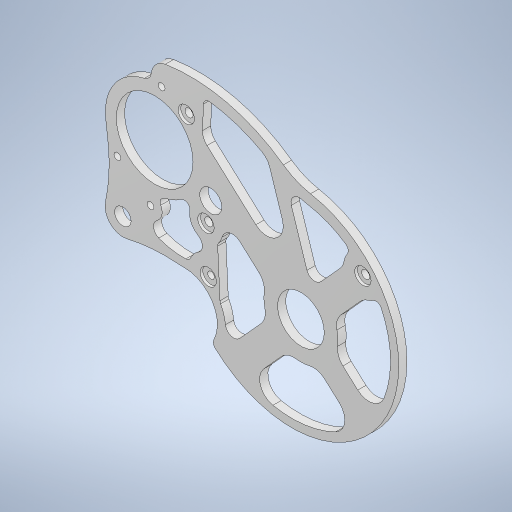
# Autodesk Inventor part: 足内フレーム
Saved by Autodesk Inventor 2023 (Build 270158000, 158)
## iProperties
Created: 2022-01-10
Part Number: 足内フレーム
Material: Aluminum 2014-T4
Document SubType Name: Modeling
Designer: acps
Density: 2.8 g/cm^3
Appearance: Satin
Author: acps
Autodesk Inventor part; units mm, degrees
ref_plane "YZ Plane" through (0, 0, 0) normal (1, 0, 0) x (0, 1, 0)
ref_plane "XZ Plane" through (0, 0, 0) normal (0, 1, 0) x (-1, 0, 0)
ref_plane "XY Plane" through (0, 0, 0) normal (0, 0, 1) x (1, 0, 0)
sketch "Sketch9" plane through (0, 0, 0) normal (0, 0, 1) x (1, 0, 0)
  circle A0 centre (46.616, 30) radius 14
  circle A1 centre (67.0906, 21) radius 20.5 construction
  arc A2 (89.1412, -35.261) -> (103.4815, 41.4054) centre (96.6972, 3) ccw
  arc A3 (28.8489, 27.1141) -> (89.1412, -35.261) centre (103.8658, 39.2989) ccw construction
  arc A4 (68.1999, -22.3859) -> (57.3086, -4.9334) centre (57.511, -16.9317) ccw
  arc A5 (68.1999, -22.3859) -> (68.6165, -24.7568) centre (69.9813, -23.2949) ccw
  arc A6 (68.6165, -24.7568) -> (89.1412, -35.261) centre (97.2785, 5.9432) ccw
  circle A7 centre (65.359, 13) radius 3
  circle A8 centre (66.1789, -3.483) radius 4 construction
  circle A9 centre (66.1789, -3.483) radius 3
  circle A10 centre (66.1789, -3.483) radius 1.25
  circle A11 centre (49.1519, 48.073) radius 1.25
  circle A12 centre (45.1, 8.5) radius 1.25
  circle A13 centre (33, 18) radius 1.25
  arc A14 (110.5809, -8.3302) -> (32.9301, 51.0574) centre (65.359, 13) ccw construction
  circle A15 centre (65.359, 13) radius 1.5
  arc A16 (116.9346, 29.0833) -> (126.4034, 19.1104) centre (122.6202, 25) ccw
  arc A17 (129.2953, 18.2763) -> (126.4034, 19.1104) centre (127.4843, 17.4276) ccw
  arc A18 (116.9346, 29.0833) -> (116.4381, 31.9015) centre (115.3101, 30.25) ccw
  circle A19 centre (67.0906, 21) radius 1.5
  circle A20 centre (67.0906, 21) radius 4.5 construction
  circle A21 centre (49.1519, 48.073) radius 4.25 construction
  arc A22 (42.888, 47.6097) -> (45.3636, 50.3845) centre (42.2376, 50.6816) ccw
  arc A23 (42.888, 47.6097) -> (28.8489, 27.1141) centre (46.616, 30) ccw
  arc A24 (50.502, 55.8582) -> (45.3636, 50.3845) centre (51.4661, 49.8045) ccw
  arc A25 (93.5981, 45.5879) -> (50.502, 55.8582) centre (59.6238, -1.42) ccw
  arc A26 (93.5981, 45.5879) -> (103.4815, 41.4054) centre (107.6564, 65.0395) ccw
  arc A27 (116.4381, 31.9015) -> (102.7857, 37.4664) centre (96.6972, 3) ccw
  arc A28 (91.2551, 42.346) -> (102.7857, 37.4664) centre (107.6564, 65.0395) ccw
  arc A29 (91.2551, 42.346) -> (66.6678, 52.1186) centre (59.6238, -1.42) ccw
  arc A30 (66.6678, 52.1186) -> (64.4084, 50.2128) centre (66.4069, 50.1357) ccw
  line L0 (64.4084, 50.2128) -> (63.6467, 30.4665)
  arc A31 (63.6467, 30.4665) -> (65.9495, 28.4127) centre (65.6452, 30.3894) ccw
  arc A32 (72.0057, 15.3351) -> (65.9495, 28.4127) centre (67.0906, 21) ccw
  arc A33 (62.3527, 39.5241) -> (63.2626, 46.965) centre (58.1571, 43.8132) ccw construction
  arc A34 (72.0057, 15.3351) -> (71.327, 13.6183) centre (73.3164, 13.8244) ccw
  arc A35 (70.0506, 9.2598) -> (71.327, 13.6183) centre (65.359, 13) ccw
  arc A36 (63.4085, 27.3516) -> (62.8815, 34.943) centre (46.616, 30) ccw construction
  arc A37 (70.0506, 9.2598) -> (69.6169, 7.9138) centre (71.6145, 8.0131) ccw
  line L1 (69.6169, 7.9138) -> (70.4543, -8.9212)
  arc A38 (70.4543, -8.9212) -> (70.6941, -9.7759) centre (72.4519, -8.8218) ccw
  arc A39 (71.6917, -21.8214) -> (70.6941, -9.7759) centre (57.511, -16.9317) ccw
  arc A40 (72.3015, -24.0094) -> (89.7225, -32.3179) centre (97.2785, 5.9432) ccw
  arc A41 (71.6917, -21.8214) -> (72.3015, -24.0094) centre (73.5824, -22.4733) ccw
  line L2 (65.359, 13) -> (66.1789, -3.483) construction
  arc A42 (89.7225, -32.3179) -> (129.2953, 18.2763) centre (96.6972, 3) ccw
  arc A43 (29.8136, 19.0227) -> (57.3086, -4.9334) centre (56.8493, 22.2958) ccw
  arc A44 (50.2005, 13.3822) -> (56.3412, 16.0565) centre (46.616, 30) ccw
  arc A45 (59.4537, 14.062) -> (56.3412, 16.0565) centre (57.4853, 14.4161) ccw
  arc A46 (47.4858, 4.9828) -> (48.8551, 10.4905) centre (45.1, 8.5) ccw
  arc A47 (59.4537, 14.062) -> (62.4846, 7.7333) centre (65.359, 13) ccw
  arc A48 (48.0848, -0.2968) -> (58.0139, -1.9093) centre (56.8493, 22.2958) ccw
  arc A49 (62.5868, 2.5251) -> (59.7536, -0.7053) centre (66.1789, -3.483) ccw
  arc A50 (58.0139, -1.9093) -> (59.7536, -0.7053) centre (57.9178, 0.0884) ccw
  arc A51 (50.2005, 13.3822) -> (48.8551, 10.4905) centre (50.6222, 11.4271) ccw
  arc A52 (62.5868, 2.5251) -> (62.4846, 7.7333) centre (61.0474, 5.1) ccw
  arc A53 (47.4858, 4.9828) -> (48.0848, -0.2968) centre (49.1698, 2.5001) ccw
  circle A54 centre (33, 18) radius 3 construction
  line L3 (29.8136, 19.0227) -> (28.7465, 27.8366)
  circle A55 centre (122.6202, 25) radius 3
  circle A56 centre (122.6202, 25) radius 1.5
  circle A57 centre (100, 0) radius 30 construction
  circle A58 centre (100, 0) radius 8.525
  circle A59 centre (100, 0) radius 13.525
  circle A60 centre (58.1571, 43.8132) radius 3
  circle A61 centre (58.1571, 43.8132) radius 1.5
  arc A62 (114.2643, 23.2173) -> (115.7252, 26.2077) centre (109.8151, 27.2429) ccw
  line L4 (114.2643, 23.2173) -> (107.1156, 15.3165)
  arc A63 (101.847, 13.3983) -> (107.1156, 15.3165) centre (102.6664, 19.3421) ccw
  line L5 (100, 0) -> (122.6202, 25) construction
  arc A64 (124.5093, 18.2597) -> (121.6794, 16.5079) centre (126.1286, 12.4824) ccw
  arc A65 (114.5307, 8.6072) -> (113.1474, 3.1737) centre (118.9799, 4.5816) ccw
  line L6 (114.5307, 8.6072) -> (121.6794, 16.5079)
  line L7 (100, 0) -> (74.2211, 23.325) construction
  arc A66 (91.3928, 14.5307) -> (96.8263, 13.1474) centre (95.4184, 18.9799) ccw
  arc A67 (86.6017, 1.847) -> (84.6835, 7.1156) centre (80.6579, 2.6664) ccw
  line L8 (77.7137, 13.4219) -> (84.6835, 7.1156)
  line L9 (91.3928, 14.5307) -> (65.7201, 37.7597)
  arc A68 (77.7137, 13.4219) -> (71.1616, 11.4735) centre (75.0299, 10.4559) ccw
  arc A69 (64.0785, 41.66) -> (65.7201, 37.7597) centre (69.0748, 41.4673) ccw
  arc A70 (108.6072, -14.5307) -> (103.1737, -13.1474) centre (104.5816, -18.9799) ccw
  arc A71 (113.3983, -1.847) -> (115.3165, -7.1156) centre (119.3421, -2.6664) ccw
  line L10 (100, 0) -> (122.2456, -20.128) construction
  line L11 (108.6072, -14.5307) -> (114.0305, -19.4378)
  line L12 (115.3165, -7.1156) -> (120.7448, -12.0272)
  arc A72 (112.6664, -29.2643) -> (114.0305, -19.4378) centre (110.0049, -23.8869) ccw
  arc A73 (120.7448, -12.0272) -> (130.3851, -9.6937) centre (124.7704, -7.5781) ccw
  arc A74 (85.4693, -8.6072) -> (86.8526, -3.1737) centre (81.0201, -4.5816) ccw
  arc A75 (98.153, -13.3983) -> (92.8844, -15.3165) centre (97.3336, -19.3421) ccw
  line L13 (85.4693, -8.6072) -> (77.655, -17.2435)
  line L14 (86.4647, -22.4117) -> (92.8844, -15.3165)
  line L15 (100, 0) -> (77.6565, -24.6942) construction
  arc A76 (72.4439, -15.5142) -> (77.655, -17.2435) centre (75.4304, -15.2307) ccw
  arc A77 (86.4647, -22.4117) -> (89.7566, -32.3246) centre (90.9138, -26.4372) ccw
  line L16 (93.2749, 27.9268) -> (88.6115, 42.3986)
  arc A78 (88.6115, 42.3986) -> (85.8103, 45.8057) centre (82.9007, 40.5584) ccw
  line L17 (102.1859, 16.5753) -> (96.489, 34.2545)
  arc A79 (100.1488, 38.0647) -> (96.489, 34.2545) centre (99.3445, 35.1746) ccw
  line L18 (91.2551, 42.346) -> (98.5171, 19.8098) construction
  arc A80 (102.1859, 16.5753) -> (107.2659, 15.4827) centre (105.0414, 17.4955) ccw
  arc A81 (83.5385, 21.6375) -> (93.2749, 27.9268) centre (87.5641, 26.0866) ccw
  circle A82 centre (67.0906, 21) radius 4.025
  circle A83 centre (35, 0) radius 3.025
  circle A84 centre (35, 0) radius 6.5
  arc A85 (28.6471, 1.3751) -> (29.7376, 19.7272) centre (-29.9949, 14.0681) ccw
  arc A86 (54.8296, -4.8623) -> (36.5033, -6.3238) centre (50.3798, -64.6971) ccw
  point P0 (0, 0)
  point P1 (0, 0)
  point P2 (89.7528, -32.3239)
  point P3 (89.7566, -32.3246)
  point P4 (29.7671, 19.4073)
  dimension "d291" = 2
  dimension "d292" = 42
  dimension "d293" = 74
  dimension "d294" = 118
  dimension "d295" = 6
  dimension "d296" = 8
  dimension "d297" = 6
  dimension "d298" = 2.5
  dimension "d299" = 2.5
  dimension "d300" = 2.5
  dimension "d301" = 8.5
  dimension "d302" = 45.1
  dimension "d303" = 2.5
  dimension "d304" = 18
  dimension "d305" = 33
  dimension "d306" = 50
  dimension "d307" = 3
  dimension "d308" = 2
  dimension "d309" = 2
  dimension "d310" = 3
  dimension "d311" = 3
  dimension "d312" = 3
  dimension "d313" = 4
  dimension "d314" = 4
  dimension "d315" = 2
  dimension "d316" = 2
  dimension "d317" = 3
  dimension "d318" = 2
  dimension "d319" = 3
  dimension "d320" = 3
  dimension "d321" = 2
  dimension "d322" = 2
  dimension "d323" = 3
  dimension "d324" = 2
  dimension "d325" = 3
  dimension "d326" = 12
  dimension "d327" = 3
  dimension "d328" = 2
  dimension "d329" = 3
  dimension "d330" = 3
  dimension "d331" = 3
  dimension "d332" = 3
  dimension "d333" = 2
  dimension "d334" = 3
  dimension "d335" = 3
  dimension "d336" = 2
  dimension "d337" = 6
  dimension "d338" = 4
  dimension "d339" = 17.05
  dimension "d340" = 5
  dimension "d341" = 3
  dimension "d342" = 6
  dimension "d343" = 6
  dimension "d344" = 5
  dimension "d345" = 6
  dimension "d346" = 6
  dimension "d347" = 10
  dimension "d348" = 6
  dimension "d349" = 6
  dimension "d350" = 10
  dimension "d351" = 5
  dimension "d352" = 4
  dimension "d353" = 5
  dimension "d354" = 6
  constraints: 141 point on circle, 85 centre point, 77 tangent, 38 end point, 14 concentric, 11 parallel, 9 coincident, 3 perpendicular, 3 point on line, 1 horizontal alignment, 39 other
  measures "d291" radius of A5
  measures "d292" radius of A6
  measures "d295" diameter of A7
  measures "d296" diameter of A8
  measures "d297" diameter of A9
  measures "d298" diameter of A10
  measures "d299" diameter of A11
  measures "d300" diameter of A12
  measures "d301" vertical distance of point (0, 0) A12.centre
  measures "d302" horizontal distance of point (0, 0) A12.centre
  measures "d303" diameter of A13
  measures "d304" vertical distance of point (0, 0) A13.centre
  measures "d305" horizontal distance of point (0, 0) A13.centre
  measures "d306" radius of A14
  measures "d307" diameter of A15
  measures "d308" radius of A17
  measures "d309" radius of A18
  measures "d310" diameter of A19
  measures "d311" radial gap between concentric circles of A19 A20
  measures "d312" radial gap between concentric circles of A11 A21
  measures "d313" radial gap between concentric circles of A27 A2
  measures "d314" radial gap between concentric circles of A28 A26
  measures "d315" radius of A30
  measures "d316" radius of A31
  measures "d317" radial gap between concentric circles of A20 A32
  measures "d318" radius of A34
  measures "d319" radial gap between concentric circles of A7 A35
  measures "d320" radial gap between concentric circles of A0 A36
  measures "d321" radius of A37
  measures "d322" radius of A38
  measures "d323" radial gap between concentric circles of A4 A39
  measures "d324" radius of A41
  measures "d325" radial gap between concentric circles of A2 A42
  measures "d326" radius of A4
  measures "d327" radial gap between concentric circles of A0 A44
  measures "d328" radius of A45
  measures "d329" radial gap between concentric circles of A12 A46
  measures "d330" radial gap between concentric circles of A7 A47
  measures "d331" radial gap between concentric circles of A43 A48
  measures "d332" radial gap between concentric circles of A49 A8
  measures "d333" radius of A51
  measures "d334" radius of A52
  measures "d335" radius of A53
  measures "d336" radius of A50
  measures "d337" diameter of A54
  measures "d338" radial gap between concentric circles of A16 A55
  measures "d339" diameter of A58
  measures "d341" radial gap between concentric circles of A33 A60
  measures "d342" radius of A62
  measures "d343" radius of A63
  measures "d344" distance between parallel lines of L5 L4
  measures "d345" radius of A64
  measures "d346" radius of A65
  measures "d347" distance between parallel lines of L4 L6
  measures "d348" radius of A66
  measures "d349" radius of A67
  measures "d350" distance between parallel lines of L8 L9
  measures "d351" distance between parallel lines of L9 L7
  measures "d352" radius of A68
  measures "d353" radius of A69
  measures "d354" radius of A70
extrude "Extrusion6" add sketch "Sketch9" along normal blind 3 contours A6 A5 A4 A43 A84 L3 A23 A22 A24 A25 A26 A2 | A86 A84 A43 | A84 A43 | A43 A84 | A84 A85 L3 A43 | A16 A64 L6 A65 A59 A63 L4 A62 | L4 A63 A59 A66 L9 A81 L16 A78 A29 A28 A79 L17 A80 | A42 A72 L11 A70 A59 A71 L12 A73 | A59 | A59 A67 L8 A68 A35 A34 A32 A31 L0 A69 L9 A66 | A40 A41 A39 A76 L13 A74 A59 A75 L14 A77
extrude "Extrusion7" add sketch "Sketch9" along normal blind 2 contours A7 | A9 | A55 | A60
sketch "Sketch10" plane through (0, 0, 3) normal (0, 0, 1) x (1, 0, 0)
  arc A0 (100.1488, 38.0647) -> (102.7857, 37.4664) centre (107.6564, 65.0395) ccw projected
  arc A1 (116.4381, 31.9015) -> (102.7857, 37.4664) centre (96.6972, 3) ccw projected
  arc A2 (116.9346, 29.0833) -> (116.4381, 31.9015) centre (115.3101, 30.25) ccw projected
  arc A3 (116.9346, 29.0833) -> (115.7252, 26.2077) centre (122.6202, 25) ccw projected
  arc A4 (114.2643, 23.2173) -> (115.7252, 26.2077) centre (109.8151, 27.2429) ccw projected
  line L0 (114.2643, 23.2173) -> (107.2659, 15.4827) projected
  arc A5 (102.1859, 16.5753) -> (107.2659, 15.4827) centre (105.0414, 17.4955) ccw projected
  line L1 (102.1859, 16.5753) -> (96.489, 34.2545) projected
  arc A6 (100.1488, 38.0647) -> (96.489, 34.2545) centre (99.3445, 35.1746) ccw projected
  arc A7 (108.6072, -14.5307) -> (103.1737, -13.1474) centre (104.5816, -18.9799) ccw projected
  line L2 (108.6072, -14.5307) -> (114.0305, -19.4378) projected
  arc A8 (112.6664, -29.2643) -> (114.0305, -19.4378) centre (110.0049, -23.8869) ccw projected
  arc A9 (89.7566, -32.3246) -> (112.6664, -29.2643) centre (96.6972, 3) ccw projected
  arc A10 (86.4647, -22.4117) -> (89.7566, -32.3246) centre (90.9138, -26.4372) ccw projected
  line L3 (86.4647, -22.4117) -> (92.8844, -15.3165) projected
  arc A11 (98.153, -13.3983) -> (92.8844, -15.3165) centre (97.3336, -19.3421) ccw projected
  arc A12 (98.153, -13.3983) -> (103.1737, -13.1474) centre (100, 0) ccw projected
  circle A13 centre (49.1519, 48.073) radius 1.25 projected
  circle A14 centre (67.0906, 21) radius 4.025 projected
  circle A15 centre (58.1571, 43.8132) radius 3 projected
  circle A16 centre (122.6202, 25) radius 3 projected
  arc A17 (47.4858, 4.9828) -> (48.8551, 10.4905) centre (45.1, 8.5) ccw projected
  arc A18 (50.2005, 13.3822) -> (48.8551, 10.4905) centre (50.6222, 11.4271) ccw projected
  arc A19 (50.2005, 13.3822) -> (56.3412, 16.0565) centre (46.616, 30) ccw projected
  arc A20 (59.4537, 14.062) -> (56.3412, 16.0565) centre (57.4853, 14.4161) ccw projected
  arc A21 (59.4537, 14.062) -> (62.4846, 7.7333) centre (65.359, 13) ccw projected
  arc A22 (62.5868, 2.5251) -> (62.4846, 7.7333) centre (61.0474, 5.1) ccw projected
  arc A23 (62.5868, 2.5251) -> (59.7536, -0.7053) centre (66.1789, -3.483) ccw projected
  arc A24 (58.0139, -1.9093) -> (59.7536, -0.7053) centre (57.9178, 0.0884) ccw projected
  arc A25 (48.0848, -0.2968) -> (58.0139, -1.9093) centre (56.8493, 22.2958) ccw projected
  arc A26 (47.4858, 4.9828) -> (48.0848, -0.2968) centre (49.1698, 2.5001) ccw projected
  circle A27 centre (33, 18) radius 1.25 projected
  circle A28 centre (45.1, 8.5) radius 1.25 projected
  circle A29 centre (66.1789, -3.483) radius 3 projected
  circle A30 centre (65.359, 13) radius 3 projected
  circle A31 centre (46.616, 30) radius 14 projected
  circle A32 centre (100, 0) radius 8.525 projected
  arc A33 (86.6017, 1.847) -> (86.8526, -3.1737) centre (100, 0) ccw projected
  arc A34 (85.4693, -8.6072) -> (86.8526, -3.1737) centre (81.0201, -4.5816) ccw projected
  line L4 (85.4693, -8.6072) -> (77.655, -17.2435) projected
  arc A35 (72.4439, -15.5142) -> (77.655, -17.2435) centre (75.4304, -15.2307) ccw projected
  arc A36 (72.4439, -15.5142) -> (70.6941, -9.7759) centre (57.511, -16.9317) ccw projected
  arc A37 (70.4543, -8.9212) -> (70.6941, -9.7759) centre (72.4519, -8.8218) ccw projected
  line L5 (70.4543, -8.9212) -> (69.6169, 7.9138) projected
  arc A38 (70.0506, 9.2598) -> (69.6169, 7.9138) centre (71.6145, 8.0131) ccw projected
  arc A39 (70.0506, 9.2598) -> (71.1616, 11.4735) centre (65.359, 13) ccw projected
  arc A40 (77.7137, 13.4219) -> (71.1616, 11.4735) centre (75.0299, 10.4559) ccw projected
  line L6 (77.7137, 13.4219) -> (84.6835, 7.1156) projected
  arc A41 (86.6017, 1.847) -> (84.6835, 7.1156) centre (80.6579, 2.6664) ccw projected
  arc A42 (114.5307, 8.6072) -> (113.1474, 3.1737) centre (118.9799, 4.5816) ccw projected
  line L7 (114.5307, 8.6072) -> (121.6794, 16.5079) projected
  arc A43 (124.5093, 18.2597) -> (121.6794, 16.5079) centre (126.1286, 12.4824) ccw projected
  arc A44 (124.5093, 18.2597) -> (126.4034, 19.1104) centre (122.6202, 25) ccw projected
  arc A45 (129.2953, 18.2763) -> (126.4034, 19.1104) centre (127.4843, 17.4276) ccw projected
  arc A46 (130.3851, -9.6937) -> (129.2953, 18.2763) centre (96.6972, 3) ccw projected
  arc A47 (120.7448, -12.0272) -> (130.3851, -9.6937) centre (124.7704, -7.5781) ccw projected
  line L8 (120.7448, -12.0272) -> (115.3165, -7.1156) projected
  arc A48 (113.3983, -1.847) -> (115.3165, -7.1156) centre (119.3421, -2.6664) ccw projected
  arc A49 (113.3983, -1.847) -> (113.1474, 3.1737) centre (100, 0) ccw projected
  arc A50 (42.888, 47.6097) -> (28.7465, 27.8366) centre (46.616, 30) ccw projected
  line L9 (28.7465, 27.8366) -> (29.7671, 19.4073) projected
  arc A51 (54.8296, -4.8623) -> (57.3086, -4.9334) centre (56.8493, 22.2958) ccw projected
  arc A52 (68.1999, -22.3859) -> (57.3086, -4.9334) centre (57.511, -16.9317) ccw projected
  arc A53 (68.1999, -22.3859) -> (68.6165, -24.7568) centre (69.9813, -23.2949) ccw projected
  arc A54 (68.6165, -24.7568) -> (89.1412, -35.261) centre (97.2785, 5.9432) ccw projected
  arc A55 (89.1412, -35.261) -> (103.4815, 41.4054) centre (96.6972, 3) ccw projected
  arc A56 (93.5981, 45.5879) -> (103.4815, 41.4054) centre (107.6564, 65.0395) ccw projected
  arc A57 (93.5981, 45.5879) -> (50.502, 55.8582) centre (59.6238, -1.42) ccw projected
  arc A58 (50.502, 55.8582) -> (45.3636, 50.3845) centre (51.4661, 49.8045) ccw projected
  arc A59 (42.888, 47.6097) -> (45.3636, 50.3845) centre (42.2376, 50.6816) ccw projected
  arc A60 (88.6115, 42.3986) -> (85.8103, 45.8057) centre (82.9007, 40.5584) ccw projected
  line L10 (88.6115, 42.3986) -> (93.2749, 27.9268) projected
  arc A61 (83.5385, 21.6375) -> (93.2749, 27.9268) centre (87.5641, 26.0866) ccw projected
  line L11 (83.5385, 21.6375) -> (65.7201, 37.7597) projected
  arc A62 (64.0785, 41.66) -> (65.7201, 37.7597) centre (69.0748, 41.4673) ccw projected
  line L12 (64.0785, 41.66) -> (64.4084, 50.2128) projected
  arc A63 (66.6678, 52.1186) -> (64.4084, 50.2128) centre (66.4069, 50.1357) ccw projected
  arc A64 (85.8103, 45.8057) -> (66.6678, 52.1186) centre (59.6238, -1.42) ccw projected
  circle A65 centre (58.1571, 43.8132) radius 1.5 projected
  circle A66 centre (65.359, 13) radius 1.5 projected
  circle A67 centre (66.1789, -3.483) radius 1.25 projected
  circle A68 centre (122.6202, 25) radius 1.5 projected
  arc A69 (28.6471, 1.3751) -> (29.7671, 19.4073) centre (-29.9949, 14.0681) ccw projected
  arc A70 (28.6471, 1.3751) -> (36.5033, -6.3238) centre (35, 0) ccw projected
  arc A71 (54.8296, -4.8623) -> (36.5033, -6.3238) centre (50.3798, -64.6971) ccw projected
  point P0 (0, 0)
body "Solid2"
